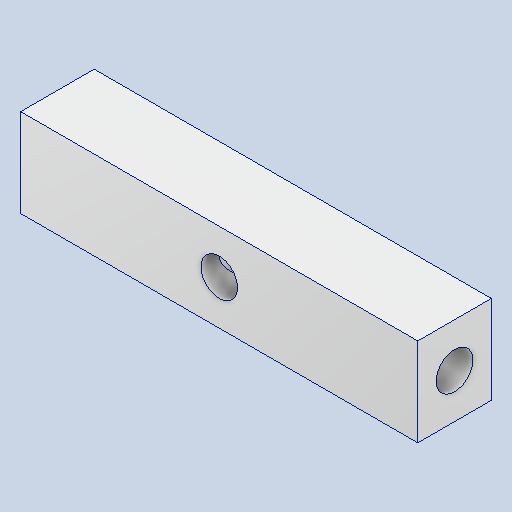
# Autodesk Inventor part: belt_liner_v5_Plate_9
Saved by Autodesk Inventor 2025.2 (Build 292293000, 293)
## iProperties
Created: 2025-01-06
Part Number: belt_liner_v5_Plate_9
Material: アルミニウム 6061
Document SubType Name: Modeling
Designer: haruy
Density: 2.7 g/cm^3
Appearance: アルミニウム - フラット
Author: haruy
Autodesk Inventor part; units mm, degrees
ref_plane "YZ Plane" through (0, 0, 0) normal (1, 0, 0) x (0, 1, 0)
ref_plane "XZ Plane" through (0, 0, 0) normal (0, 1, 0) x (-1, 0, 0)
sketch "スケッチ1" plane through (0, 0, 0) normal (1, 0, 0) x (0, 1, 0)
  line L0 (0, 0) -> (6, 0)
  line L1 (6, 0) -> (6, -5)
  line L2 (6, -5) -> (0, -5)
  line L3 (0, -5) -> (0, 0)
  point P0 (3, -2.5)
  dimension "d0" = 6
  dimension "d1" = 5
  dimension "d2" = 3
  dimension "d3" = 2.5
  constraints: 8 end point, 2 parallel, 1 horizontal, 1 perpendicular
  measures "d0" distance of L1.end L2.end
  measures "d1" distance of L0.end L1.end
  measures "d2" distance from line of point (3, -2.5) L1
  measures "d3" distance from line of point (3, -2.5) L0
extrude "押し出し1" add sketch "スケッチ1" against normal blind 27
ref_plane "作業平面1" through (-29.5, 0, 0) normal (1, 0, 0) x (0, 0, -1)
hole "穴1" at (0, 3, -2.5) direction (-1, 0, 0) diameter 2.5 end through all
sketch "スケッチ3" plane through (0, 0, -5) normal (0, 0, -1) x (-1, 0, 0)
  line L0 (0, 0) -> (27, 0) projected
  line L1 (0, 0) -> (0, 6) projected
  point P0 (13.5, 3)
  dimension "d19" = 3
  dimension "d20" = 13.5
  measures "d19" distance from line of point (13.5, 3) L0
  measures "d20" distance from line of L1 point (13.5, 3)
hole "穴2" at (-13.5, 3, -5) direction (0, 0, 1) diameter 2.5 end through all
